Autodesk Fusion 360 part; units mm, degrees
note: some values were not read from the file. Chosen so that the rebuilt part matches the saved one: which face or edge a step refers to. Set by a fixed rule: which sketch regions a step uses.
(part 2 of 2)
sketch "Skizze27" plane through (194, 0, 0) normal (1, 0, 0) x (0, 1, 0)
  circle A0 centre (-87.6878, -32) radius 2
  circle A1 centre (-64.3937, 32) radius 2
  line L0 (-65.0684, 46.8121) -> (-99.1448, -46.8121)
  line L1 (-99.1448, -46.8121) -> (-87.0132, -46.8121)
  line L2 (-87.0132, -46.8121) -> (-52.9368, 46.8121)
  line L3 (-52.9368, 46.8121) -> (-65.0684, 46.8121)
  circle A2 centre (-64.3937, 32) radius 1.6
  circle A3 centre (-87.6878, -32) radius 1.6
  line L4 (-99.1448, -46.8121) -> (-39.1448, -46.8121)
  line L5 (-39.1448, -46.8121) -> (-39.1448, -41.8121)
  line L6 (-39.1448, -41.8121) -> (-99.1448, -41.8121)
  line L7 (-99.1448, -41.8121) -> (-99.1448, -46.8121)
  circle A4 centre (-64.3937, 32) radius 4
  circle A5 centre (-87.6878, -32) radius 4
  line L8 (-90.2057, -46.8121) -> (-57.2212, 43.8121)
  line L9 (-57.2212, 43.8121) -> (-62.9678, 43.8121)
  line L10 (-62.9678, 43.8121) -> (-95.9523, -46.8121)
  line L11 (-94.8604, -43.8121) -> (-89.1138, -43.8121)
  dimension "d212" = 3.2
  dimension "d213" = 3.2
  dimension "d214" = 5
  dimension "d215" = 60
  dimension "d216" = 8
  dimension "d217" = 8
  constraint concentric A1 A2
  constraint concentric A0 A3
  constraint horizontal L4
  constraint vertical L5
  constraint horizontal L6
  constraint vertical L7
  constraint concentric A2 A4
  constraint concentric A3 A5
  constraint parallel L2 L8
  constraint parallel L3 L9
  constraint parallel L0 L10
  constraint parallel L1 L11
  constraint coincident L0.end L1.start
  constraint coincident L1 L10.end
  constraint coincident L11.start L10
  constraint coincident L1 L8.start
  constraint coincident L11.end L8
  measures "d212" diameter of A2
  measures "d213" diameter of A3
  measures "d214" distance of L0.end L6.end
  measures "d215" distance of L5.end L6.end
  measures "d216" diameter of A4
  measures "d217" diameter of A5
extrude "Extrusion41" add sketch "Skizze27" along normal blind 12 separate body contours A0 | A1 | L6 A5 L8 L10 | L6 L8 L10 L11 | L2 L4 L5 L6 | L1 L2 L4 L6 L8 | L1 L4 L8 L10 L11 | A5 L8 L10 | A5 L10 | A5 L8 | A4 A5 L8 L10 | A4 L8 L10 | A4 L10 | A4 L8 | A4 L8 L9 L10 makes body 16
fillet "Abrundung1" radius 62.5 1 edges at (200, -88.3859, -41.8121) on bodies 16
fillet "Abrundung2" radius 7.5 1 edges at (200, -86.1601, -35.6967) on bodies 16
sketch "Skizze28" plane through (0, 0, 65) normal (0, 0, 1) x (-1, 0, 0)
  circle A0 centre (-152.7, 28.4485) radius 1.6
  circle A1 centre (-187.7, 28.4485) radius 1.6
  circle A2 centre (-172.2, 27.5985) radius 7
  line L0 (-141.4667, -65) -> (-141.4667, -47)
  line L1 (-141.4667, -47) -> (-70.7333, -47)
  line L2 (-70.7333, -47) -> (-70.7333, -65)
  line L3 (-70.7333, -65) -> (0, -65)
  line L4 (0, -65) -> (0, -23.8505)
  line L5 (0, -23.8505) -> (-18, -23.8505)
  line L6 (-18, -23.8505) -> (-18, 17.299)
  line L7 (-18, 17.299) -> (0, 17.299)
  line L8 (0, 17.299) -> (0, 58.4485)
  line L9 (0, 58.4485) -> (-212.2, 58.4485)
  line L10 (-212.2, 58.4485) -> (-212.2, 17.299)
  line L11 (-212.2, 17.299) -> (-194.2, 17.299)
  line L12 (-194.2, 17.299) -> (-194.2, -23.8505)
  line L13 (-194.2, -23.8505) -> (-212.2, -23.8505)
  line L14 (-212.2, -23.8505) -> (-212.2, -65)
  line L15 (-212.2, -65) -> (-141.4667, -65)
  circle A3 centre (-152.7, 28.4485) radius 1.6
  circle A4 centre (-136.1325, 28.4485) radius 1.6
  circle A5 centre (-114.1325, 28.4485) radius 1.6
  circle A6 centre (-125.1325, 28.4485) radius 4.6
  dimension "d225" = 3.2
  dimension "d226" = 3.2
  dimension "d227" = 9.2
  dimension "d228" = 22
  dimension "d229" = 11
  constraint horizontal A4.centre A6.centre
  measures "d225" diameter of A4
  measures "d226" diameter of A5
  measures "d227" diameter of A6
  measures "d228" distance of A4.centre A5.centre
  measures "d229" distance of A4.centre A6.centre
extrude "Extrusion42" cut sketch "Skizze28" against normal blind 18 contours A4 | A5 | A6 bodies 4
sketch "Skizze29" plane through (0, 65, 0) normal (0, 1, 0) x (-1, 0, 0)
  line L0 (-18, 21.6667) -> (0, 21.6667)
  line L1 (0, 21.6667) -> (0, 47)
  line L2 (0, 47) -> (-70.7333, 47)
  line L3 (-70.7333, 47) -> (-70.7333, 65)
  line L4 (-70.7333, 65) -> (-141.4667, 65)
  line L5 (-141.4667, 65) -> (-141.4667, 47)
  line L6 (-141.4667, 47) -> (-212.2, 47)
  line L7 (-212.2, 47) -> (-212.2, 21.6667)
  line L8 (-212.2, 21.6667) -> (-194.2, 21.6667)
  line L9 (-194.2, 21.6667) -> (-194.2, -21.6667)
  line L10 (-194.2, -21.6667) -> (-212.2, -21.6667)
  line L11 (-212.2, -21.6667) -> (-212.2, -47)
  line L12 (-212.2, -47) -> (-141.4667, -47)
  line L13 (-141.4667, -47) -> (-141.4667, -65)
  line L14 (-141.4667, -65) -> (-70.7333, -65)
  line L15 (-70.7333, -65) -> (-70.7333, -47)
  line L16 (-70.7333, -47) -> (0, -47)
  line L17 (0, -47) -> (0, -21.6667)
  line L18 (0, -21.6667) -> (-18, -21.6667)
  line L19 (-18, -21.6667) -> (-18, 21.6667)
  circle A0 centre (-171, 39.5) radius 1.6
  circle A1 centre (-171, -39.5) radius 1.6
  circle A2 centre (-171, 21.5) radius 12.1
  circle A3 centre (-171, -21.5) radius 12.1
  line L20 (-183.1, 21.5) -> (-183.1, -21.5)
  line L21 (-158.9, 21.5) -> (-158.9, -21.5)
  dimension "d232" = 3.2
  dimension "d233" = 3.2
  dimension "d234" = 79
  dimension "d235" = 7.5
  dimension "d236" = 7.5
  dimension "d237" = 24.2
  dimension "d238" = 18
  dimension "d239" = 24.2
  dimension "d240" = 18
  constraint vertical A0.centre A1.centre
  constraint vertical A0.centre A2.centre
  constraint vertical A1.centre A3.centre
  constraint coincident A2 L20.start
  constraint coincident A3 L20.end
  constraint tangent A3 L20
  constraint vertical L20
  constraint coincident A2 L21.start
  constraint coincident A3 L21.end
  constraint tangent A3 L21
  constraint vertical L21
  measures "d232" diameter of A0
  measures "d233" diameter of A1
  measures "d234" distance of A0.centre A1.centre
  measures "d235" distance of L6 A0.centre
  measures "d236" distance of L12 A1.centre
  measures "d237" diameter of A2
  measures "d238" distance of A0.centre A2.centre
  measures "d239" diameter of A3
  measures "d240" distance of A1.centre A3.centre
extrude "Extrusion43" cut sketch "Skizze29" against normal blind 18 contours A0 | A1 | A2 | A2 A3 L20 L21 | A3 bodies 3
sketch "Skizze30" plane through (0, 0, 65) normal (0, 0, 1) x (-1, 0, 0)
  circle A0 centre (-114.1325, 28.4485) radius 1.6
  circle A1 centre (-125.1325, 28.4485) radius 4.6
  circle A2 centre (-136.1325, 28.4485) radius 1.6
  circle A3 centre (-152.7, 28.4485) radius 1.6
  circle A4 centre (-187.7, 28.4485) radius 1.6
  circle A5 centre (-172.2, 27.5985) radius 7
  line L0 (-141.4667, -65) -> (-141.4667, -47)
  line L1 (-141.4667, -47) -> (-70.7333, -47)
  line L2 (-70.7333, -47) -> (-70.7333, -65)
  line L3 (-70.7333, -65) -> (0, -65)
  line L4 (0, -65) -> (0, -23.8505)
  line L5 (0, -23.8505) -> (-18, -23.8505)
  line L6 (-18, -23.8505) -> (-18, 17.299)
  line L7 (-18, 17.299) -> (0, 17.299)
  line L8 (0, 17.299) -> (0, 58.4485)
  line L9 (0, 58.4485) -> (-212.2, 58.4485)
  line L10 (-212.2, 58.4485) -> (-212.2, 17.299)
  line L11 (-212.2, 17.299) -> (-194.2, 17.299)
  line L12 (-194.2, 17.299) -> (-194.2, -23.8505)
  line L13 (-194.2, -23.8505) -> (-212.2, -23.8505)
  line L14 (-212.2, -23.8505) -> (-212.2, -65)
  line L15 (-212.2, -65) -> (-141.4667, -65)
  line L16 (-212.2, 65) -> (-212.2, 58.4485)
  line L17 (-212.2, 58.4485) -> (0, 58.4485)
  line L18 (0, 58.4485) -> (0, 65)
  line L19 (0, 65) -> (-212.2, 65)
  line L20 (0, 58.4485) -> (-212.2, 58.4485)
  line L21 (-212.2, 58.4485) -> (-212.2, 81.3623)
  line L22 (-212.2, 81.3623) -> (0, 81.3623)
  line L23 (0, 81.3623) -> (0, 58.4485)
  constraint horizontal L20
  constraint vertical L21
  constraint horizontal L22
  constraint vertical L23
  constraint coincident L8.end L9.start
ref_plane "Arbeitsebene5" through (106.1, -17.1066, 0) normal (1, 0, 0) x (0, -1, 0)
sketch "Skizze31" plane through (0, 65, 0) normal (0, 1, 0) x (-1, 0, 0)
  arc A0 (-183.1, -21.5) -> (-158.9, -21.5) centre (-171, -21.5) ccw
  line L0 (-183.1, -21.5) -> (-183.1, 21.5)
  arc A1 (-158.9, 21.5) -> (-183.1, 21.5) centre (-171, 21.5) ccw
  line L1 (-158.9, 21.5) -> (-158.9, -21.5)
  circle A2 centre (-171, 39.5) radius 1.6
  circle A3 centre (-171, -39.5) radius 1.6
  line L2 (-18, 21.6667) -> (0, 21.6667)
  line L3 (0, 21.6667) -> (0, 47)
  line L4 (0, 47) -> (-70.7333, 47)
  line L5 (-70.7333, 47) -> (-70.7333, 65)
  line L6 (-70.7333, 65) -> (-141.4667, 65)
  line L7 (-141.4667, 65) -> (-141.4667, 47)
  line L8 (-141.4667, 47) -> (-212.2, 47)
  line L9 (-212.2, 47) -> (-212.2, 21.6667)
  line L10 (-212.2, 21.6667) -> (-194.2, 21.6667)
  line L11 (-194.2, 21.6667) -> (-194.2, -21.6667)
  line L12 (-194.2, -21.6667) -> (-212.2, -21.6667)
  line L13 (-212.2, -21.6667) -> (-212.2, -47)
  line L14 (-212.2, -47) -> (-141.4667, -47)
  line L15 (-141.4667, -47) -> (-141.4667, -65)
  line L16 (-141.4667, -65) -> (-70.7333, -65)
  line L17 (-70.7333, -65) -> (-70.7333, -47)
  line L18 (-70.7333, -47) -> (0, -47)
  line L19 (0, -47) -> (0, -21.6667)
  line L20 (0, -21.6667) -> (-18, -21.6667)
  line L21 (-18, -21.6667) -> (-18, 21.6667)
  line L22 (-119.1, 15) -> (-93.1, 15)
  line L23 (-93.1, 15) -> (-93.1, 7)
  line L24 (-93.1, 7) -> (-119.1, 7)
  line L25 (-119.1, 7) -> (-119.1, 15)
  line L26 (0, 65) -> (-212.2, 65)
  circle A4 centre (-85.5, 11) radius 1.6
  circle A5 centre (-126.7, 11) radius 1.6
  point P0 (-106.1, 65)
  point P1 (-106.1, 15)
  point P2 (-93.1, 11)
  dimension "d243" = 26
  dimension "d244" = 8
  dimension "d245" = 50
  dimension "d246" = 3.2
  dimension "d247" = 3.2
  dimension "d248" = 41.2
  dimension "d249" = 20.6
  constraint horizontal L22
  constraint vertical L23
  constraint horizontal L24
  constraint vertical L25
  constraint midpoint L6 P0
  constraint midpoint L22 P1
  constraint vertical P0 P1
  constraint midpoint L23 P2
  measures "d243" distance of L22.start L22.end
  measures "d244" distance of L22.start L24.end
  measures "d245" distance of L22 L26
  measures "d246" diameter of A4
  measures "d247" diameter of A5
  measures "d248" distance of A4.centre A5.centre
  measures "d249" horizontal distance of P1 A4.centre
extrude "Extrusion44" cut sketch "Skizze31" against normal up to surface (18 mm away) contours L22 L23 L24 L25 | A4 | A5 bodies 3
sketch "Skizze32" plane through (0, 0, 65) normal (0, 0, 1) x (-1, 0, 0)
  circle A0 centre (-114.1325, 28.4485) radius 1.6
  circle A1 centre (-125.1325, 28.4485) radius 4.6
  circle A2 centre (-136.1325, 28.4485) radius 1.6
  circle A3 centre (-152.7, 28.4485) radius 1.6
  circle A4 centre (-187.7, 28.4485) radius 1.6
  circle A5 centre (-172.2, 27.5985) radius 7
  line L0 (-141.4667, -65) -> (-141.4667, -47)
  line L1 (-141.4667, -47) -> (-70.7333, -47)
  line L2 (-70.7333, -47) -> (-70.7333, -65)
  line L3 (-70.7333, -65) -> (0, -65)
  line L4 (0, -65) -> (0, -23.8505)
  line L5 (0, -23.8505) -> (-18, -23.8505)
  line L6 (-18, -23.8505) -> (-18, 17.299)
  line L7 (-18, 17.299) -> (0, 17.299)
  line L8 (0, 17.299) -> (0, 58.4485)
  line L9 (0, 58.4485) -> (-212.2, 58.4485)
  line L10 (-212.2, 58.4485) -> (-212.2, 17.299)
  line L11 (-212.2, 17.299) -> (-194.2, 17.299)
  line L12 (-194.2, 17.299) -> (-194.2, -23.8505)
  line L13 (-194.2, -23.8505) -> (-212.2, -23.8505)
  line L14 (-212.2, -23.8505) -> (-212.2, -65)
  line L15 (-212.2, -65) -> (-141.4667, -65)
  circle A6 centre (-114.1325, 28.4485) radius 1.6
  circle A7 centre (-125.1325, 28.4485) radius 4.6
  circle A8 centre (-136.1325, 28.4485) radius 1.6
  circle A9 centre (-114.1325, 28.4485) radius 3.6
  circle A10 centre (-136.1325, 28.4485) radius 3.6
  circle A11 centre (-125.1325, 28.4485) radius 7.5
  circle A12 centre (-125.1325, 28.4485) radius 4.25
  circle A13 centre (-152.7, 28.4485) radius 3.6
  circle A14 centre (-187.7, 28.4485) radius 3.6
  circle A15 centre (-172.2, 27.5985) radius 9.9
  line L16 (-152.7013, 24.8485) -> (-187.7, 24.8485)
  line L17 (-187.7, 32.0485) -> (-152.7, 32.0485)
  dimension "d252" = 7.2
  dimension "d253" = 7.2
  dimension "d254" = 15
  dimension "d261" = 8.5
  dimension "d262" = 7.2
  dimension "d263" = 7.2
  dimension "d264" = 2.9
  constraint concentric A0 A9
  constraint concentric A2 A10
  constraint concentric A7 A11
  constraint concentric A1 A12
  constraint concentric A3 A13
  constraint concentric A4 A14
  constraint coincident A13 L16.start
  constraint coincident A14 L16.end
  constraint tangent A14 L16
  constraint horizontal L16
  constraint coincident A14 L17.start
  constraint coincident A13 L17.end
  constraint tangent A13 L17
  constraint horizontal L17
  measures "d252" diameter of A9
  measures "d253" diameter of A10
  measures "d254" diameter of A11
  measures "d261" diameter of A12
  measures "d262" diameter of A13
  measures "d263" diameter of A14
extrude "Extrusion45" add sketch "Skizze32" along normal blind 1 separate body contours A1 A7 | A9 A11 | A9 A11 | A9 A10 A11 | A10 A11 | A10 A11 makes body 17
fillet "Abrundung3" radius 7 4 edges at (117.6648, -29.1436, 65.5) (117.6648, -27.7535, 65.5) (132.6003, -29.1436, 65.5) (132.6003, -27.7535, 65.5) on bodies 17
hidden bodies 1 2 15 16 17
equation "d62 = d61"
equation "d68 = d67"
equation "d118 = 123.448536 mm / 3"
equation "d120 = d118"
equation "d132 = 123.448536 mm / 3"
equation "d133 = d132"
equation "d139 = 164.213202 mm / 3"
equation "d140 = d139"
equation "d146 = 164.213202 mm / 3"
equation "d147 = d146"
equation "d153 = 212.20 mm / 3"
equation "d154 = d153"
equation "d164 = 130.00 mm / 3"
equation "d165 = d164"
equation "d204 = d203"
named bodies: "Left", "Bottom", "Back", "Top", "Right", "Keyboard Plate", "PCB"
